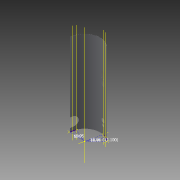
# Autodesk Inventor part: EDM Middle Shield Part 1
Saved by Autodesk Inventor 2015 (Build 190159000, 159)
## iProperties
Created: 2014-06-18
Part Number: EDM Middle Shield Part 1
Material: Generic
Document SubType Name: Modeling
Designer: Aki
Density: 1 g/cm^3
Appearance: Default
Sheet Metal Rule: Default
Author: Aki
Autodesk Inventor part; units mm, degrees
ref_plane "YZ Plane" through (0, 0, 0) normal (1, 0, 0) x (0, 1, 0)
ref_plane "XZ Plane" through (0, 0, 0) normal (0, 1, 0) x (-1, 0, 0)
ref_plane "XY Plane" through (0, 0, 0) normal (0, 0, 1) x (1, 0, 0)
sketch "Sketch4" plane through (0, 0, 0) normal (0, 1, 0) x (-1, 0, 0)
  arc A0 (-218.1621, -216.479) -> (307.0256, -13.8983) centre (0, 0) ccw
  line L0 (0, 0) -> (-218.1621, -216.479) construction
  line L1 (0, 0) -> (307.0256, -13.8983) construction
  arc A1 (-217.2606, -215.5845) -> (305.7569, -13.8408) centre (0, 0) ccw
  line L2 (0, 0) -> (-217.2606, -215.5845) construction
  line L3 (0, 0) -> (305.7569, -13.8408) construction
  line L4 (307.0256, -13.8983) -> (305.7569, -13.8408)
  line L5 (-218.1621, -216.479) -> (-217.2606, -215.5845)
  dimension "d14" = 307.34
  dimension "d15" = 132.63
  dimension "d16" = 306.07
  dimension "d17" = 132.63
  constraints: 12 end point, 4 point on circle, 2 centre point, 2 coincident, 1 collinear, 1 point on line
  measures "d14" radius of A0
  measures "d15" angle of L0 L1
  measures "d16" radius of A1
  measures "d17" angle of L2 L3
extrude "Extrusion1" add sketch "Sketch4" along normal blind 1625.6
sketch "Sketch6" plane through (0, 0, 0) normal (0, 1, 0) x (-1, 0, 0)
  arc A0 (-218.1621, -216.479) -> (-64.2241, -300.5547) centre (0, 0) ccw
  line L0 (0, 0) -> (-64.2241, -300.5547) construction
  line L1 (0, 0) -> (-218.1621, -216.479) construction
  arc A1 (-218.1621, -216.479) -> (-136.0382, -275.593) centre (0, 0) ccw
  line L2 (0, 0) -> (-136.0382, -275.593) construction
  line L3 (0, 0) -> (-218.1621, -216.479) construction
  arc A2 (285.8722, -112.8494) -> (307.0256, -13.8983) centre (0, 0) ccw
  line L4 (0, 0) -> (285.8722, -112.8494) construction
  line L5 (0, 0) -> (307.0256, -13.8983) construction
  dimension "d22" = 33.16
  dimension "d64" = 307.34
  dimension "d65" = 18.95
  dimension "d66" = 18.95
  constraints: 12 end point, 6 point on circle, 3 centre point, 3 coincident
  measures "d22" angle of L1 L0
  measures "d64" radius of A1
  measures "d65" angle of L3 L2
  measures "d66" angle of L4 L5
ref_plane "Work Plane3" through (64.2241, 0, -300.5547) normal (0.2089677, 0, -0.9779225) x (0, 1, 0)
sketch "Sketch7" plane through (64.2241, 0, -300.5547) normal (0.2089677, 0, -0.9779225) x (0, 1, 0)
  circle A0 centre (158.75, 0) radius 25.4
  point P0 (0, 0)
  dimension "d23" = 158.75
  dimension "d24" = 50.8
  constraints: 1 centre point
  measures "d23" distance of point (0, 0) A0.centre
  measures "d24" diameter of A0
hole "Hole1" at (64.2241, 158.75, -300.5547) direction (-0.2089677, 0, 0.9779225) diameter 50.8 end through all
sketch "Sketch8" plane through (64.2241, 0, -300.5547) normal (0.2089677, 0, -0.9779225) x (0, 1, 0)
  circle A0 centre (238.125, 0) radius 38.1
  point P0 (0, 0)
  dimension "d32" = 76.2
  dimension "d33" = 238.125
  constraints: 1 centre point
  measures "d32" diameter of A0
  measures "d33" distance of point (0, 0) A0.centre
hole "Hole2" at (64.2241, 238.125, -300.5547) direction (-0.2089677, 0, 0.9779225) diameter 76.2 end through all
sketch "Sketch9" plane through (64.2241, 0, -300.5547) normal (0.2089677, 0, -0.9779225) x (0, 1, 0)
  circle A0 centre (871.5375, 0) radius 38.1
  line L0 (0, -307.34) -> (0, 168.1085) projected
  point P0 (0, 0)
  point P1 (0, -303.1515)
  dimension "d41" = 76.2
  dimension "d42" = 871.5375
  constraints: 1 centre point
  measures "d41" diameter of A0
  measures "d42" distance from line of L0 A0.centre
hole "Hole3" at (64.2241, 871.5375, -300.5547) direction (-0.2089677, 0, 0.9779225) diameter 76.2 end through all
sketch "Sketch10" plane through (64.2241, 0, -300.5547) normal (0.2089677, 0, -0.9779225) x (0, 1, 0)
  circle A0 centre (1019.175, 0) radius 63.5
  line L0 (0, 167.4138) -> (0, -306.07) projected
  point P0 (0, 0)
  point P1 (0, -301.8988)
  dimension "d50" = 127
  dimension "d51" = 1019.175
  constraints: 1 centre point
  measures "d50" diameter of A0
  measures "d51" distance from line of L0 A0.centre
hole "Hole4" at (64.2241, 1019.175, -300.5547) direction (-0.2089677, 0, 0.9779225) diameter 127 end through all
sketch "Sketch11" plane through (0, 0, 0) normal (0, 1, 0) x (-1, 0, 0)
  arc A0 (300.5547, -64.2241) -> (307.0256, -13.8983) centre (0, 0) ccw
  line L0 (0, 0) -> (300.5547, -64.2241) construction
  line L1 (0, 0) -> (307.0256, -13.8983) construction
  dimension "d59" = 9.47
  constraints: 4 end point, 2 point on circle, 1 centre point, 1 coincident
  measures "d59" angle of L0 L1
ref_plane "Work Plane4" through (-300.5547, 0, -64.2241) normal (-0.9779225, 0, -0.2089677) x (0, -1, 0)
sketch "Sketch12" plane through (-300.5547, 0, -64.2241) normal (-0.9779225, 0, -0.2089677) x (0, -1, 0)
  circle A0 centre (-158.75, 0) radius 88.9
  line L0 (0, 50.567) -> (0, -307.34) projected
  line L1 (-247.65, 0) -> (-69.85, 0)
  line L2 (-69.85, 0) -> (-69.85, 88.9)
  line L3 (-69.85, 88.9) -> (-247.65, 88.9)
  line L4 (-247.65, 88.9) -> (-247.65, 0)
  point P0 (0, 0)
  point P1 (0, -257.2886)
  dimension "d60" = 177.8
  dimension "d61" = 158.75
  constraints: 8 end point, 2 parallel, 1 horizontal, 1 horizontal alignment, 1 perpendicular, 2 other
  measures "d61" distance from line of L0 point (-158.75, 0)
extrude "Extrusion2" cut sketch "Sketch12" against normal blind 25.4
equation "\"BendRadius\" = Thickness"
equation "\"BendReliefWidth\" = Thickness"
equation "\"BendReliefDepth\" = 0.5 * Thickness"
equation "\"CornerReliefSize\" = 4 * Thickness"
equation "\"MinimumRemnant\" = 2 * Thickness"
equation "\"TransitionRadius\" = BendRadius"
equation "\"JacobiRadiusSize\" = Thickness"
equation "\"GapSize\" = Thickness"
equation "\"Thickness\" = 3.048"
body "Solid1"
